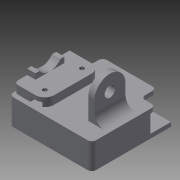
# Autodesk Inventor part: MotorHolder_NOPCB
Saved by Autodesk Inventor 2014 SP1 (Build 180222100, 222)
## iProperties
Created: 2013-11-09
Part Number: MotorHolder_NOPCB
Material: Generic
Document SubType Name: Modeling
Designer: JustinIndra
Density: 1 g/cm^3
Appearance: Default
Author: JustinIndra
Autodesk Inventor part; units mm, degrees
ref_plane "YZ Plane" through (0, 0, 0) normal (1, 0, 0) x (0, 1, 0)
sketch "Sketch1" plane through (0, 0, 0) normal (0, 1, 0) x (-1, 0, 0)
  line L0 (20, 0) -> (-20, 0)
  line L1 (-20, 0) -> (-20, 10)
  line L2 (-20, 10) -> (20, 10)
  line L3 (20, 10) -> (20, 0)
  circle A0 centre (0, 0) radius 3.175
  arc A1 (-20, 0) -> (20, 0) centre (0, 16.3026) ccw
  line L4 (20, 0) -> (-20, 0)
  line L5 (13.2784, -9.5) -> (-17.2645, -9.5) construction
  line L6 (20, 10) -> (-20, 10)
  line L7 (-20, 10) -> (-20, -10)
  line L8 (-20, -10) -> (20, -10)
  line L9 (20, -10) -> (20, 10)
  dimension "d0" = 40
  dimension "d2" = 6.35
  dimension "d4" = 9.5
  dimension "d5" = 10
  dimension "d6" = 20
  constraints: 20 end point, 5 parallel, 3 coincident, 3 perpendicular, 2 centre point, 2 horizontal, 2 point on circle, 1 collinear, 1 midpoint, 1 tangent
  measures "d0" distance of L1.end L2.end
  measures "d2" diameter of A0
  measures "d4" distance between parallel lines of L5 L0
  measures "d5" distance of L0.end L1.end
  measures "d6" distance of L8.end L2.end
extrude "Extrusion1" add sketch "Sketch1" along normal mid plane 8.5 contours L9 L8 L7 A1
sketch "Sketch2" plane through (0, -4.25, 0) normal (0, -1, 0) x (1, 0, 0)
  line L0 (20, -10) -> (20, 0) projected
  line L1 (-20, -10) -> (20, -10)
  line L2 (20, -10) -> (20, 10)
  line L3 (20, 10) -> (-20, 10)
  line L4 (-20, 10) -> (-20, -10)
  point P0 (0, 0)
  dimension "d9" = 20
  constraints: 8 end point, 2 parallel, 1 collinear, 1 horizontal, 1 perpendicular
  measures "d9" distance of L3.end L1.start
extrude "Extrusion2" add sketch "Sketch2" along normal blind 2
sketch "Sketch4" plane through (0, -4.25, 0) normal (0, 1, 0) x (1, 0, 0)
  circle A0 centre (0, 0) radius 3.175
  dimension "d12" = 6.35
  constraints: 1 centre point, 1 coincident
  measures "d12" diameter of A0
extrude "Extrusion3" cut sketch "Sketch4" against normal through all
mirror "Mirror1" about plane through (0, 0, 0) normal (0, 1, 0) of "Extrusion2", "Extrusion3"
sketch "Sketch5" plane through (0, -6.25, 0) normal (0, -1, 0) x (1, 0, 0)
  line L0 (-20, -10) -> (20, -10) projected
  line L1 (-20, 10) -> (-13, 10)
  line L2 (-13, 10) -> (-13, 2.5)
  line L3 (-13, 2.5) -> (-20, 2.5)
  line L4 (-20, 2.5) -> (-20, 10)
  dimension "d15" = 7
  dimension "d17" = 12.5
  constraints: 8 end point, 2 parallel, 1 horizontal, 1 perpendicular
  measures "d15" distance of L2.end L3.end
  measures "d17" distance between parallel lines of L3 L0
extrude "Extrusion4" cut sketch "Sketch5" against normal up to next
mirror "Mirror2" about plane through (0, 0, 0) normal (1, 0, 0) of "Extrusion4"
sketch "Sketch6" plane through (20, -6.25, -10) normal (0, 0, -1) x (-1, 0, 0)
  line L0 (40, 0) -> (40, 12.5) projected
  line L1 (0, 0) -> (40, 0)
  line L2 (40, 0) -> (40, 12.5)
  line L3 (40, 12.5) -> (0, 12.5)
  line L4 (0, 12.5) -> (0, 0)
  point P0 (20, 6.25)
  dimension "d20" = 12.5
  constraints: 8 end point, 2 parallel, 1 horizontal, 1 perpendicular, 1 point on line
  measures "d20" distance of L3.end L1.start
extrude "Extrusion5" add sketch "Sketch6" along normal blind 18.25
sketch "Sketch7" plane through (0, -6.25, 0) normal (0, -1, 0) x (1, 0, 0)
  circle A0 centre (0, 0) radius 3.175 projected
  line L0 (-7.5, -5) -> (-4.5, -5)
  line L1 (-4.5, -5) -> (-4.5, -20)
  line L2 (-4.5, -20) -> (-7.5, -20)
  line L3 (-7.5, -20) -> (-7.5, -5)
  line L4 (10, -5) -> (13, -5)
  line L5 (13, -5) -> (13, -20)
  line L6 (13, -20) -> (10, -20)
  line L7 (10, -20) -> (10, -5)
  dimension "d23" = 15
  dimension "d25" = 3
  dimension "d26" = 4.5
  dimension "d27" = 5
  dimension "d28" = 14.5
  constraints: 16 end point, 4 parallel, 2 equal length, 2 horizontal, 2 perpendicular, 1 collinear
  measures "d23" distance of L2.end L0.start
  measures "d25" distance of L1.end L2.end
  measures "d26" distance from line of A0.centre L1
  measures "d27" distance from line of A0.centre L0
  measures "d28" distance between parallel lines of L1 L7
extrude "Extrusion6" add sketch "Sketch7" along normal blind 17.5 contours L4 L5 L6 L7
sketch "Sketch8" plane through (10, -6.25, -20) normal (-1, 0, 0) x (0, 0, 1)
  line L0 (15, -17.5) -> (0, -17.5)
  circle A0 centre (7.5, -10) radius 2.55
  line L1 (0, 0) -> (15, 0) projected
  line L2 (0, 0) -> (0, -17.5) projected
  line L3 (15, -17.5) -> (0, -17.5) projected
  line L4 (15, 0) -> (15, -17.5) projected
  point P0 (20, 6.25)
  point P1 (7.5, -17.5)
  dimension "d31" = 5.1
  dimension "d34" = 7.5
  constraints: 2 end point, 1 centre point, 1 midpoint, 1 vertical alignment
  measures "d31" diameter of A0
  measures "d34" distance from line of L0 A0.centre
extrude "Extrusion7" cut sketch "Sketch8" against normal through all contours A0
fillet "Fillet1" radius 7.5 2 edges at (11.5, -23.75, -5) (11.5, -23.75, -20)
sketch "Sketch9" plane through (0, -6.25, 0) normal (0, -1, 0) x (1, 0, 0)
  line L0 (10, -20) -> (10, -5) projected
  line L1 (-20, 1) -> (-5, 1)
  line L2 (-5, 1) -> (-5, -26)
  line L3 (-5, -26) -> (-20, -26)
  line L4 (-20, -26) -> (-20, 1)
  line L5 (-20, 2.5) -> (-20, -28.25) projected
  point P0 (-5, -12.5)
  point P1 (10, -12.5)
  dimension "d38" = 15
  dimension "d39" = 27
  constraints: 8 end point, 2 midpoint, 2 parallel, 1 collinear, 1 horizontal, 1 horizontal alignment, 1 perpendicular
  measures "d38" distance between parallel lines of L0 L2
  measures "d39" distance of L3.end L1.start
extrude "Extrusion8" add sketch "Sketch9" along normal blind 4
ref_plane "Work Plane1" through (0, -8.25, 0) normal (0, -1, 0) x (1, 0, 0)
sketch "Sketch10" plane through (0, -8.25, 0) normal (0, -1, 0) x (1, 0, 0)
  line L0 (-7, -4.9434) -> (-9.5, -6.3868)
  line L1 (-9.5, -6.3868) -> (-12, -4.9434)
  line L2 (-12, -4.9434) -> (-12, -2.0566)
  line L3 (-12, -2.0566) -> (-9.5, -0.6132)
  line L4 (-9.5, -0.6132) -> (-7, -2.0566)
  line L5 (-7, -2.0566) -> (-7, -4.9434)
  line L6 (-5, -26) -> (-5, 1) projected
  line L7 (-5, -12.5) -> (-18.5359, -12.5) construction
  line L8 (-12, -3.5) -> (-7, -3.5)
  line L9 (-7, -3.5) -> (-7, 1)
  line L10 (-7, 1) -> (-12, 1)
  line L11 (-12, 1) -> (-12, -3.5)
  line L12 (-5, 1) -> (-20, 1) projected
  point P0 (0, 0)
  point P1 (-9.5, -3.5)
  dimension "d44" = 5
  dimension "d45" = 4.5
  dimension "d46" = 9
  constraints: 22 end point, 2 collinear, 2 midpoint, 2 parallel, 2 perpendicular, 1 horizontal, 1 vertical, 13 other
  measures "d44" distance between parallel lines of L5 L2
  measures "d45" distance from line of L6 point (-9.5, -3.5)
  measures "d46" distance from line of L7 point (-9.5, -3.5)
extrude "Extrusion9" cut sketch "Sketch10" against normal blind 2
ref_plane "Work Plane2" through (-20, -10.25, -12.5) normal (0, 0, 1) x (1, 0, 0)
mirror "Mirror3" about plane through (-20, -10.25, -12.5) normal (0, 0, 1) of "Extrusion9"
sketch "Sketch11" plane through (0, -10.25, 0) normal (0, -1, 0) x (1, 0, 0)
  line L0 (-20, 1) -> (-20, -26) projected
  line L1 (-5, -26) -> (-5, 1) projected
  line L2 (-5, -12.5) -> (-20, -12.5) construction
  point P0 (0, 0)
  point P1 (-9.5, -3.5)
  point P2 (-9.5, -21.5)
  dimension "d49" = 4.5
  dimension "d50" = 18
  constraints: 2 end point, 2 midpoint, 1 symmetric about line
  measures "d49" distance from line of L1 point (-9.5, -3.5)
  measures "d50" distance of point (-9.5, -21.5) point (-9.5, -3.5)
hole "Hole1" at (-9.5, -10.25, -3.5) at (-9.5, -10.25, -21.5) direction (0, 1, 0) diameter 2.013 depth 4 tip angle 118 thread size "M2.5x0.45" class "6H" standard "ISO Metric profile"
sketch "Sketch12" plane through (-20, -4.25, 0) normal (-1, 0, 0) x (0, 0, 1)
  line L0 (-7.5, -6) -> (-17.5, -6)
  line L1 (-17.5, -6) -> (-17.5, -12)
  line L2 (-17.5, -12) -> (-7.5, -12)
  line L3 (-7.5, -12) -> (-7.5, -6)
  line L4 (1, -6) -> (-26, -6) projected
  point P0 (-26, -6.25)
  point P1 (-12.5, -12)
  point P2 (-12.5, -6)
  dimension "d58" = 6
  dimension "d61" = 10
  constraints: 8 end point, 2 midpoint, 2 parallel, 1 collinear, 1 horizontal, 1 perpendicular, 1 vertical alignment
  measures "d58" distance of L0.end L1.end
  measures "d61" distance of L1.end L2.end
extrude "Extrusion10" add sketch "Sketch12" against normal blind 4
sketch "Sketch13" plane through (-20, -6.25, -26) normal (-1, 0, 0) x (0, 0, -1)
  line L0 (-8.5, 10) -> (-18.5, 10) projected
  circle A0 centre (-13.5, 10) radius 6
  point P0 (-26, -6.25)
  dimension "d64" = 12
  constraints: 1 centre point, 1 midpoint
  measures "d64" diameter of A0
extrude "Extrusion11" cut sketch "Sketch13" against normal blind 5
sketch "Sketch14" plane through (-20, -10.25, -7.5) normal (0, 0, 1) x (1, 0, 0)
  line L0 (0, -2.6834) -> (4, -2.6834) projected
  line L1 (4, 0) -> (4, -2.6834) projected
  line L2 (0, 0) -> (4, 0) projected
  line L3 (0, -2.6834) -> (0, 0) projected
  point P0 (20, 10.25)
extrude "Extrusion12" add sketch "Sketch14" along normal blind 2
mirror "Mirror4" about plane through (-20, -10.25, -12.5) normal (0, 0, 1) of "Extrusion12"
fillet "Fillet2" radius 4.5 2 edges at (-5, -8.25, 1) (-5, -8.25, -26)
fillet "Fillet3" radius 5 1 edges at (13, -6.25, -12.5)
fillet "Fillet4" radius 2 9 edges at (-13, -5.25, 10) (-13, -5.25, 2.5) (13, -5.25, 10) (13, -5.25, 2.5) (20, -5.25, 2.5) (-20, -5.25, 2.5) (20, 0, -28.25) (-20, 0, -28.25) (-20, -8.25, -26)
equation "\"d6\" = 2 * d5"
body "Solid1"
